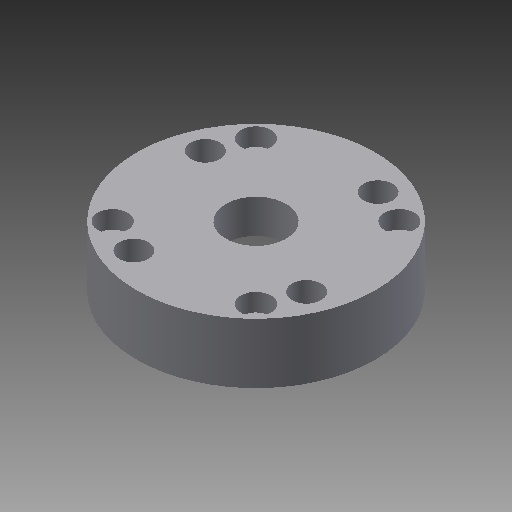
# Autodesk Inventor part: 09-1NT-0.125-FO1_BM_heads-bif
Saved by Autodesk Inventor 2019.4 (Build 234330000, 330)
## iProperties
Category: PARTsolutions
Company: BIMBA
Created: 2020-02-04
Part Number: 09-1NT-0.125-FO1_BM_heads-bif
Material: Generic
Catalog Web Link: www.cadenas.de
Description: FO1 Basic Model Heads-Bimba FLAT-1
Vendor: BIMBA
Document SubType Name: Modeling
Designer: psadmin
Manufacturer: BIMBA
Mass: 18.4876 g
Surface Area: 81.253 cm^2
Volume: 18.4876 cm^3
Density: 1 g/cm^3
Appearance: PSOLRGB-211-211-211
PSOL_IDENT_0: {$CADENAS_DATA\23d-libs\bimba\bimba_brand\bimba_imperial\bimba_full_line\flat_cylinders\fo1\fo1_basi
PSOL_IDENT_1: c_model_heads_right.prj},268 {VTYP=3D},{NB=09-1NT-0.125-FO1_BM_heads-bif},{LINA=09-1NT-0.125-FO1_BM_
PSOL_IDENT_2: heads-bif},{NN=FO1 Basic Model Heads},{DATE=22.01.2020 09:06:03},{GEOMDATE=10.10.2019 07:16:13},{VER
PSOL_IDENT_3: SION=},{LINEID=30},{WBVAR=MNT,LRR,ER,RTX,HD,STPT1,STPT2,STPT3,STPT4,PP,MRS,RL1},{WBNUMERIC=RL1}  {NB=
PSOL_IDENT_4: 09-1NT-0.125-FO1_BM_heads-bif},{LINA=09-1NT-0.125-FO1_BM_heads-bif},{KT=DUMMY},{PN=09-1NT-0.125-FO1_
PSOL_IDENT_5: BM_heads},{BORE=1.06250000},{BOREPN=09},{MNT=},{MNTALG='','Standard Counterbored Mounting Holes','1'
PSOL_IDENT_6: ,'Pivot Mount','1N','Pivot Mount 90 Deg. from Standard','2','[2] Trunnion Mount','3R','Threaded Moun
PSOL_IDENT_7: ting Holes, Rear','4R','Screw Clearance Holes, Rear','5','Front Nose Mount [5]','6','F Series Interc
PSOL_IDENT_8: hange, Counterbored, Rear [6]' ,'7R','F Series Interchange, Threaded, Rear [7R]'},{LRR=1},{ER=},{RTX=
PSOL_IDENT_9: NT},{RTXALG='', 'Standard', 'CFT', 'Coarse Female Thread', 'CMT'  , 'Male Rod Thread (Coarse)','MT',
PSOL_IDENT_10: 'Male Rod End (Fine)', 'NT'  , 'Non-Threaded Rod'},{HD=},{STPT1=},{STPT2=},{STPT3=},{STPT4=},{PP=},
PSOL_IDENT_11: {MRS=},{PPALG='','Standard','P2','Port Position #2','P3','Port Position #3','P4','Port Position #4'}
PSOL_IDENT_12: ,{A=1.98800000},{C=1.68800000},{AR=1.69000000},{DD=4.00000000},{D=0.13800000},{CPIL=0.15600000},{DC=
PSOL_IDENT_13: 0.25000000},{DCP=0.14800000},{DCD=1.68700000},{ES=0.31250000},{EC=0.31250000},{ED=0.70000000},{F=0.5
PSOL_IDENT_14: 0000000},{H=0.44000000},{J=0.5},{J1=0.50000000},{K=0.28},{K1=0.28000000},{K2=0.44000000},{L=0.405000
PSOL_IDENT_15: 00},{LDP=0.35500000},{LP=0.12500000},{LPDP=0.51000000},{TD=1.12200000},{TDDP=0.21800},{LSF=0.0000000
PSOL_IDENT_16: 0},{LSFDP=0.00000000},{AA=0.13000000},{AB=1.50000000},{AC=0.75000000},{AD=1.00000000},{AD1=UNS},{AE=
PSOL_IDENT_17: 0.99750000},{AF=0.55000000},{M=0.50000000},{N=0.25000000},{P=0.25000000},{Q=0.19000000},{QQ=0.252},{
PSOL_IDENT_18: R=0.13800000},{S=0.37500000},{T=0.25000000},{U=0.25000000},{W=0.81200000},{X=0.25000000},{Y=0.750000
PSOL_IDENT_19: 00},{Z=0.19000000},{A13=0.13800000},{A14=0.25000000},{ANGLE=45.00000000},{JY=0.5},{JH=0.5},{PANGLE=0
PSOL_IDENT_20: },{ANGLE1=67.5},{ANGLE11=67.50000000},{D11=0.156},{CONX=0.25000000},{CONY=0.20000000},{G=0.07000000}
PSOL_IDENT_21: ,{HH=0.55000000},{RD=0.27200000},{HDADD1=0.19000000},{HDADD=0},{GW=0.1095},{GD=0.8905},{GR=0.0460},{
PSOL_IDENT_22: PW=0.1300},{PD=0.9975},{PR=0.0150},{RL1=0.12500},{CS=1.55600},{DS=0.15400},{DCS=0.24200},{DCSP=0.180
PSOL_IDENT_23: 00},{C4=1.68800},{CD=1.68800},{C6=1.68800},{D6=0.20400},{DC6=0.37500},{DC6P=0.20000},{C7=1.68800},{R
PSOL_IDENT_24: 7=0.19000},{RC=1.55600},{RT=0.138},{RCB=0.15000},{RCD=0.10000},{PB1=0.000},{PB2=0.0000},{JB=0.302},{
PSOL_IDENT_25: AP=1.9900},{PCB=0.2500},{PCD=0.1560},{PCBD=0.145},{ALPH=65},{BDIA=0.900},{BD=0.058},{MNTRG=},{L5=1.2
PSOL_IDENT_26: 50},{NDM5=1.000},{A5=0.13000},{NANG=22.5},{UNANG=7.500}
NN: FO1 Basic Model Heads
NT: Bimba FLAT-1
NB: 09-1NT-0.125-FO1_BM_heads-bif
NBSYN: $PN.-bif
LINA: 09-1NT-0.125-FO1_BM_heads-bif
PN: 09-1NT-0.125-FO1_BM_heads
BORE: 0
BOREPN: 09
MNT: Standard Counterbored Mounting Holes
LRR: 1
ER: Single Rod
RTX: Non-Threaded Rod
HD: Standard Rear Head
STPT1: Without T1
STPT2: Without T2
STPT3: Without T3
STPT4: Without T4
PP: Standard
MRS: Without -Z
A: 1.988
C: 1.688
AR: 1.69
DD: 4
D: 0.138
CPIL: 0.156
DC: 0.25
DCP: 0.148
DCD: 1.687
ES: 0.3125
EC: 0.3125
ED: 0.7
F: 0.5
H: 0.44
J1: 0.5
K1: 0.28
K2: 0.44
L: 0.405
LDP: 0.355
LP: 0.125
LPDP: 0.51
TD: 1.122
TDDP: 0.218
LSF: 0
LSFDP: 0
AA: 0.13
AB: 1.5
AC: 0.75
AD: 1
AD1: UNS
AE: 0.9975
AF: 0.55
M: 0.5
N: 0.25
P: 0.25
Q: 0.19
QQ: 0.252
R: 0.138
S: 0.375
T: 0.25
U: 0.25
W: 0.812
X: 0.25
Y: 0.75
Z: 0.19
A13: 0.138
A14: 0.25
ANGLE: 45
ANGLE11: 67.5
CONX: 0.25
CONY: 0.2
G: 0.07
HH: 0.55
RD: 0.272
HDADD1: 0.19
GW: 0.1095
GD: 0.8905
GR: 0.046
PW: 0.13
PD: 0.9975
PR: 0.015
RL1: 0.125
CS: 1.556
DS: 0.154
DCS: 0.242
DCSP: 0.18
C4: 1.688
C6: 1.688
D6: 0.204
DC6: 0.375
DC6P: 0.2
C7: 1.688
R7: 0.19
RC: 1.556
RT: 0.138
RCB: 0.15
RCD: 0.1
PB1: 0
PB2: 0
AP: 1.99
PCB: 0.25
PCD: 0.156
PCBD: 0.145
BDIA: 0.9
BD: 0.058
L5: 1.25
NDM5: 1
A5: 0.13
NANG: 22.5
UNANG: 7.5
SUPPLIER: BIMBA
ARTICLENO: 09-1NT-0.125-FO1_BM_heads-bif
BOMINFO: 09-1NT-0.125-FO1_BM_heads-bif
CREATOR: CADENAS GmbH
Title: 09-1NT-0.125-FO1_BM_heads-bif
Author: Cadenas PARTsolutions
Comments: Bimba FLAT-1
Autodesk Inventor part; units mm, degrees
sketch "Sketch_1" plane through (0, 0, 0) normal (0, 0, 1) x (1, 0, 0)
  line L0 (0, 0) -> (0, 12.7)
  line L1 (0, 12.7) -> (25.2476, 12.7)
  line L2 (25.2476, 12.7) -> (25.2476, 0)
  line L3 (25.2476, 0) -> (0, 0)
  line L4 (0, 0) -> (0, 12.7)
  constraints: 10 end point
revolve "Revolution1" add sketch "Sketch_1" angle 360 about axis through (0, 0, 0) along (0, -1, 0)
sketch "Sketch_84" plane through (0, 0, 0) normal (0, 0, 1) x (1, 0, 0)
  line L0 (-16.2306, 5.588) -> (-25.2476, 5.588)
  line L1 (-25.2476, 5.588) -> (-25.2476, 11.0427)
  line L2 (-25.2476, 11.0427) -> (-24.6126, 10.4077)
  line L3 (-24.6126, 10.4077) -> (-16.2306, 10.146)
  line L4 (-16.2306, 10.146) -> (-16.2306, 5.588)
  line L5 (-16.2306, 5.588) -> (-25.2476, 5.588)
  constraints: 12 end point
revolve "Revolution2" cut sketch "Sketch_84" angle 360 about axis through (-16.2306, 5.588, 0) along (1, 0, 0)
thread "Thread1" size "1/8" designation "1/8 - 27 NPT" standard "NPT" full length
sketch "Sketch_85" plane through (0, 0, 0) normal (0, 0, 1) x (1, 0, 0)
  line L0 (-12.2936, 7.6708) -> (-25.2476, 7.6708)
  line L1 (-25.2476, 7.6708) -> (-25.2476, 9.2583)
  line L2 (-25.2476, 9.2583) -> (-13.2101, 9.2583)
  line L3 (-13.2101, 9.2583) -> (-12.2936, 7.6708)
  line L4 (-12.2936, 7.6708) -> (-25.2476, 7.6708)
  constraints: 10 end point
revolve "Revolution3" cut sketch "Sketch_85" angle 360 about axis through (-12.2936, 7.6708, 0) along (1, 0, 0)
sketch "Sketch4" plane through (0, 12.7, 0) normal (0, 1, 0) x (1, 0, 0)
  point P0 (-15.1587, 15.1587)
hole "Hole1" at (-15.1587, 12.7, -15.1587) direction (0, -1, 0) diameter 3.9624 depth 12.7 counterbore diameter 6.35 counterbore depth 3.7592
sketch "Sketch5" plane through (0, 12.7, 0) normal (0, 1, 0) x (1, 0, 0)
  point P0 (-15.1587, -15.1587)
hole "Hole2" at (-15.1587, 12.7, 15.1587) direction (0, -1, 0) diameter 3.9624 depth 12.7 counterbore diameter 6.35 counterbore depth 3.7592
sketch "Sketch6" plane through (0, 12.7, 0) normal (0, 1, 0) x (1, 0, 0)
  point P0 (15.1587, -15.1587)
hole "Hole3" at (15.1587, 12.7, 15.1587) direction (0, -1, 0) diameter 3.9624 depth 12.7 counterbore diameter 6.35 counterbore depth 3.7592
sketch "Sketch7" plane through (0, 12.7, 0) normal (0, 1, 0) x (1, 0, 0)
  point P0 (15.1587, 15.1587)
hole "Hole4" at (15.1587, 12.7, -15.1587) direction (0, -1, 0) diameter 3.9624 depth 12.7 counterbore diameter 6.35 counterbore depth 3.7592
sketch "Sketch8" plane through (0, 0, 0) normal (0, -1, 0) x (1, 0, 0)
  point P0 (0, 0)
hole "Hole5" at (0, 0, 0) direction (0, 1, 0) diameter 12.7508 depth 12.7
sketch "Sketch_9" plane through (0, 0, 0) normal (0, 0, 1) x (1, 0, 0)
  line L0 (0, 0) -> (0, 5.5372)
  line L1 (0, 5.5372) -> (14.2494, 5.5372)
  line L2 (14.2494, 5.5372) -> (14.2494, 0)
  line L3 (14.2494, 0) -> (0, 0)
  line L4 (0, 0) -> (0, 5.5372)
  constraints: 10 end point
revolve "Revolution4" cut sketch "Sketch_9" angle 360 about axis through (0, 0, 0) along (0, -1, 0)
sketch "Sketch10" plane through (0, 12.7, 0) normal (0, 1, 0) x (1, 0, 0)
  point P0 (-18.257, 7.5623)
hole "Hole6" at (-18.257, 12.7, -7.5623) direction (0, -1, 0) diameter 3.9116 depth 12.7 counterbore diameter 6.1468 counterbore depth 4.572
pattern_linear "Rectangular Pattern1" count 2 spacing 27.9466 along (0.9239, 0, -0.3827) count 2 spacing 27.9466 along (0.3827, 0, 0.9239) of "Hole6"
ref_plane "a1_XY" through (0, 12.7, -25.2476) normal (0, 1, 0) x (1, 0, 0)
ref_plane "a1_YZ" through (0, 12.7, -25.2476) normal (1, 0, 0) x (0, 0, -1)
ref_plane "a1_ZX" through (0, 12.7, -25.2476) normal (0, 0, -1) x (0, 1, 0)
ref_plane "a2_XY" through (0, 12.7, 25.2476) normal (0, 1, 0) x (1, 0, 0)
ref_plane "a2_YZ" through (0, 12.7, 25.2476) normal (1, 0, 0) x (0, 0, -1)
ref_plane "a2_ZX" through (0, 12.7, 25.2476) normal (0, 0, -1) x (0, 1, 0)
ref_plane "ab_tr1_XY" through (-12.9439, 0, -1.7041) normal (0, 1, 0) x (1, 0, 0)
ref_plane "ab_tr1_YZ" through (-12.9439, 0, -1.7041) normal (1, 0, 0) x (0, 0, -1)
ref_plane "ab_tr1_ZX" through (-12.9439, 0, -1.7041) normal (0, 0, -1) x (0, 1, 0)
ref_plane "ab_tr2_XY" through (12.9439, 0, 1.7041) normal (0, 1, 0) x (1, 0, 0)
ref_plane "ab_tr2_YZ" through (12.9439, 0, 1.7041) normal (1, 0, 0) x (0, 0, -1)
ref_plane "ab_tr2_ZX" through (12.9439, 0, 1.7041) normal (0, 0, -1) x (0, 1, 0)
ref_plane "ab_tr3_XY" through (-1.7041, 0, 12.9439) normal (0, 1, 0) x (1, 0, 0)
ref_plane "ab_tr3_YZ" through (-1.7041, 0, 12.9439) normal (1, 0, 0) x (0, 0, -1)
ref_plane "ab_tr3_ZX" through (-1.7041, 0, 12.9439) normal (0, 0, -1) x (0, 1, 0)
ref_plane "ab_tr4_XY" through (1.7041, 0, -12.9439) normal (0, 1, 0) x (1, 0, 0)
ref_plane "ab_tr4_YZ" through (1.7041, 0, -12.9439) normal (1, 0, 0) x (0, 0, -1)
ref_plane "ab_tr4_ZX" through (1.7041, 0, -12.9439) normal (0, 0, -1) x (0, 1, 0)
ref_plane "ar3_XY" through (-8.2135, 5.5372, 19.8292) normal (0, 1, 0) x (1, 0, 0)
ref_plane "ar3_YZ" through (-8.2135, 5.5372, 19.8292) normal (1, 0, 0) x (0, 0, -1)
ref_plane "ar3_ZX" through (-8.2135, 5.5372, 19.8292) normal (0, 0, -1) x (0, 1, 0)
ref_plane "ar4_XY" through (19.8292, 5.5372, 8.2135) normal (0, 1, 0) x (1, 0, 0)
ref_plane "ar4_YZ" through (19.8292, 5.5372, 8.2135) normal (1, 0, 0) x (0, 0, -1)
ref_plane "ar4_ZX" through (19.8292, 5.5372, 8.2135) normal (0, 0, -1) x (0, 1, 0)
ref_plane "ar5_XY" through (8.2135, 5.5372, -19.8292) normal (0, 1, 0) x (1, 0, 0)
ref_plane "ar5_YZ" through (8.2135, 5.5372, -19.8292) normal (1, 0, 0) x (0, 0, -1)
ref_plane "ar5_ZX" through (8.2135, 5.5372, -19.8292) normal (0, 0, -1) x (0, 1, 0)
ref_plane "ar6_XY" through (-19.8292, 5.5372, -8.2135) normal (0, 1, 0) x (1, 0, 0)
ref_plane "ar6_YZ" through (-19.8292, 5.5372, -8.2135) normal (1, 0, 0) x (0, 0, -1)
ref_plane "ar6_ZX" through (-19.8292, 5.5372, -8.2135) normal (0, 0, -1) x (0, 1, 0)
ref_plane "b1_XY" through (0, 12.7, 0) normal (0, 1, 0) x (1, 0, 0)
ref_plane "b1_YZ" through (0, 12.7, 0) normal (1, 0, 0) x (0, 0, -1)
ref_plane "b1_ZX" through (0, 12.7, 0) normal (0, 0, -1) x (0, 1, 0)
ref_plane "c11_XY" through (-15.1587, 12.7, -15.1587) normal (0, 1, 0) x (1, 0, 0)
ref_plane "c11_YZ" through (-15.1587, 12.7, -15.1587) normal (1, 0, 0) x (0, 0, -1)
ref_plane "c11_ZX" through (-15.1587, 12.7, -15.1587) normal (0, 0, -1) x (0, 1, 0)
ref_plane "c22_XY" through (15.1587, 12.7, 15.1587) normal (0, 1, 0) x (1, 0, 0)
ref_plane "c22_YZ" through (15.1587, 12.7, 15.1587) normal (1, 0, 0) x (0, 0, -1)
ref_plane "c22_ZX" through (15.1587, 12.7, 15.1587) normal (0, 0, -1) x (0, 1, 0)
ref_plane "d11_XY" through (-16.5596, 12.7, -13.7578) normal (0, 1, 0) x (1, 0, 0)
ref_plane "d11_YZ" through (-16.5596, 12.7, -13.7578) normal (1, 0, 0) x (0, 0, -1)
ref_plane "d11_ZX" through (-16.5596, 12.7, -13.7578) normal (0, 0, -1) x (0, 1, 0)
ref_plane "d22_XY" through (-13.7578, 12.7, -16.5596) normal (0, 1, 0) x (1, 0, 0)
ref_plane "d22_YZ" through (-13.7578, 12.7, -16.5596) normal (1, 0, 0) x (0, 0, -1)
ref_plane "d22_ZX" through (-13.7578, 12.7, -16.5596) normal (0, 0, -1) x (0, 1, 0)
ref_plane "j_XY" through (0, 0, 0) normal (0, 1, 0) x (1, 0, 0)
ref_plane "j_YZ" through (0, 0, 0) normal (1, 0, 0) x (0, 0, -1)
ref_plane "j_ZX" through (0, 0, 0) normal (0, 0, -1) x (0, 1, 0)
ref_plane "k1_XY" through (-25.2476, 5.588, 0) normal (0, 0, 1) x (1, 0, 0)
ref_plane "k1_YZ" through (-25.2476, 5.588, 0) normal (1, 0, 0) x (0, 1, 0)
ref_plane "k1_ZX" through (-25.2476, 5.588, 0) normal (0, 1, 0) x (0, 0, 1)
ref_plane "k2_XY" through (-25.2476, 12.7, 0) normal (0, 0, 1) x (1, 0, 0)
ref_plane "k2_YZ" through (-25.2476, 12.7, 0) normal (1, 0, 0) x (0, 1, 0)
ref_plane "k2_ZX" through (-25.2476, 12.7, 0) normal (0, 1, 0) x (0, 0, 1)
ref_plane "nut_XY" through (0, 26.9875, 0) normal (0, 1, 0) x (1, 0, 0)
ref_plane "nut_YZ" through (0, 26.9875, 0) normal (1, 0, 0) x (0, 0, -1)
ref_plane "nut_ZX" through (0, 26.9875, 0) normal (0, 0, -1) x (0, 1, 0)
ref_plane "po1_XY" through (18.257, 0, 7.5623) normal (0, 1, 0) x (1, 0, 0)
ref_plane "po1_YZ" through (18.257, 0, 7.5623) normal (1, 0, 0) x (0, 0, -1)
ref_plane "po1_ZX" through (18.257, 0, 7.5623) normal (0, 0, -1) x (0, 1, 0)
ref_plane "po2_XY" through (7.5623, 0, -18.257) normal (0, 1, 0) x (1, 0, 0)
ref_plane "po2_YZ" through (7.5623, 0, -18.257) normal (1, 0, 0) x (0, 0, -1)
ref_plane "po2_ZX" through (7.5623, 0, -18.257) normal (0, 0, -1) x (0, 1, 0)
ref_plane "po3_XY" through (-18.257, 0, -7.5623) normal (0, 1, 0) x (1, 0, 0)
ref_plane "po3_YZ" through (-18.257, 0, -7.5623) normal (1, 0, 0) x (0, 0, -1)
ref_plane "po3_ZX" through (-18.257, 0, -7.5623) normal (0, 0, -1) x (0, 1, 0)
ref_plane "po4_XY" through (-7.5623, 0, 18.257) normal (0, 1, 0) x (1, 0, 0)
ref_plane "po4_YZ" through (-7.5623, 0, 18.257) normal (1, 0, 0) x (0, 0, -1)
ref_plane "po4_ZX" through (-7.5623, 0, 18.257) normal (0, 0, -1) x (0, 1, 0)
ref_plane "r7_XY" through (2.413, 12.7, 21.4376) normal (0, 1, 0) x (1, 0, 0)
ref_plane "r7_YZ" through (2.413, 12.7, 21.4376) normal (1, 0, 0) x (0, 0, -1)
ref_plane "r7_ZX" through (2.413, 12.7, 21.4376) normal (0, 0, -1) x (0, 1, 0)
ref_plane "r71_XY" through (0, 12.7, 21.4376) normal (0, 1, 0) x (1, 0, 0)
ref_plane "r71_YZ" through (0, 12.7, 21.4376) normal (1, 0, 0) x (0, 0, -1)
ref_plane "r71_ZX" through (0, 12.7, 21.4376) normal (0, 0, -1) x (0, 1, 0)
ref_plane "r72_XY" through (-2.413, 12.7, 21.4376) normal (0, 1, 0) x (1, 0, 0)
ref_plane "r72_YZ" through (-2.413, 12.7, 21.4376) normal (1, 0, 0) x (0, 0, -1)
ref_plane "r72_ZX" through (-2.413, 12.7, 21.4376) normal (0, 0, -1) x (0, 1, 0)
ref_plane "r73_XY" through (0, 12.7, -21.4376) normal (0, 1, 0) x (1, 0, 0)
ref_plane "r73_YZ" through (0, 12.7, -21.4376) normal (1, 0, 0) x (0, 0, -1)
ref_plane "r73_ZX" through (0, 12.7, -21.4376) normal (0, 0, -1) x (0, 1, 0)
ref_plane "rg_XY" through (0, 12.7, 0) normal (0, 1, 0) x (1, 0, 0)
ref_plane "rg_YZ" through (0, 12.7, 0) normal (1, 0, 0) x (0, 0, -1)
ref_plane "rg_ZX" through (0, 12.7, 0) normal (0, 0, -1) x (0, 1, 0)
ref_plane "rh_XY" through (0, 12.7, 0) normal (0, 1, 0) x (1, 0, 0)
ref_plane "rh_YZ" through (0, 12.7, 0) normal (1, 0, 0) x (0, 0, -1)
ref_plane "rh_ZX" through (0, 12.7, 0) normal (0, 0, -1) x (0, 1, 0)
ref_plane "rs_1_XY" through (-15.1587, 15.2908, -15.1587) normal (0, 1, 0) x (1, 0, 0)
ref_plane "rs_1_YZ" through (-15.1587, 15.2908, -15.1587) normal (1, 0, 0) x (0, 0, -1)
ref_plane "rs_1_ZX" through (-15.1587, 15.2908, -15.1587) normal (0, 0, -1) x (0, 1, 0)
ref_plane "rs_2_XY" through (-15.1587, 15.2908, 15.1587) normal (0, 1, 0) x (1, 0, 0)
ref_plane "rs_2_YZ" through (-15.1587, 15.2908, 15.1587) normal (1, 0, 0) x (0, 0, -1)
ref_plane "rs_2_ZX" through (-15.1587, 15.2908, 15.1587) normal (0, 0, -1) x (0, 1, 0)
ref_plane "rs_3_XY" through (15.1587, 15.2908, 15.1587) normal (0, 1, 0) x (1, 0, 0)
ref_plane "rs_3_YZ" through (15.1587, 15.2908, 15.1587) normal (1, 0, 0) x (0, 0, -1)
ref_plane "rs_3_ZX" through (15.1587, 15.2908, 15.1587) normal (0, 0, -1) x (0, 1, 0)
ref_plane "rs_4_XY" through (15.1587, 15.2908, -15.1587) normal (0, 1, 0) x (1, 0, 0)
ref_plane "rs_4_YZ" through (15.1587, 15.2908, -15.1587) normal (1, 0, 0) x (0, 0, -1)
ref_plane "rs_4_ZX" through (15.1587, 15.2908, -15.1587) normal (0, 0, -1) x (0, 1, 0)
ref_plane "sc1_XY" through (7.5623, 8.128, -18.257) normal (0, 1, 0) x (1, 0, 0)
ref_plane "sc1_YZ" through (7.5623, 8.128, -18.257) normal (1, 0, 0) x (0, 0, -1)
ref_plane "sc1_ZX" through (7.5623, 8.128, -18.257) normal (0, 0, -1) x (0, 1, 0)
ref_plane "sc2_XY" through (-18.257, 8.128, -7.5623) normal (0, 1, 0) x (1, 0, 0)
ref_plane "sc2_YZ" through (-18.257, 8.128, -7.5623) normal (1, 0, 0) x (0, 0, -1)
ref_plane "sc2_ZX" through (-18.257, 8.128, -7.5623) normal (0, 0, -1) x (0, 1, 0)
ref_plane "sc3_XY" through (-7.5623, 8.128, 18.257) normal (0, 1, 0) x (1, 0, 0)
ref_plane "sc3_YZ" through (-7.5623, 8.128, 18.257) normal (1, 0, 0) x (0, 0, -1)
ref_plane "sc3_ZX" through (-7.5623, 8.128, 18.257) normal (0, 0, -1) x (0, 1, 0)
ref_plane "sc4_XY" through (18.257, 8.128, 7.5623) normal (0, 1, 0) x (1, 0, 0)
ref_plane "sc4_YZ" through (18.257, 8.128, 7.5623) normal (1, 0, 0) x (0, 0, -1)
ref_plane "sc4_ZX" through (18.257, 8.128, 7.5623) normal (0, 0, -1) x (0, 1, 0)
ref_plane "to_dummy_XY" through (0, 12.7, 0) normal (0, 1, 0) x (1, 0, 0)
ref_plane "to_dummy_YZ" through (0, 12.7, 0) normal (1, 0, 0) x (0, 0, -1)
ref_plane "to_dummy_ZX" through (0, 12.7, 0) normal (0, 0, -1) x (0, 1, 0)
ref_plane "to_nut_XY" through (0, 16.002, 0) normal (0, 1, 0) x (1, 0, 0)
ref_plane "to_nut_YZ" through (0, 16.002, 0) normal (1, 0, 0) x (0, 0, -1)
ref_plane "to_nut_ZX" through (0, 16.002, 0) normal (0, 0, -1) x (0, 1, 0)
ref_plane "to_rod_XY" through (0, 0, 0) normal (0, 1, 0) x (1, 0, 0)
ref_plane "to_rod_YZ" through (0, 0, 0) normal (1, 0, 0) x (0, 0, -1)
ref_plane "to_rod_ZX" through (0, 0, 0) normal (0, 0, -1) x (0, 1, 0)
ref_plane "to_tube_XY" through (0, 5.5372, 0) normal (0, 1, 0) x (1, 0, 0)
ref_plane "to_tube_YZ" through (0, 5.5372, 0) normal (1, 0, 0) x (0, 0, -1)
ref_plane "to_tube_ZX" through (0, 5.5372, 0) normal (0, 0, -1) x (0, 1, 0)
ref_plane "to_wiper_XY" through (0, 12.7, 0) normal (0, 1, 0) x (1, 0, 0)
ref_plane "to_wiper_YZ" through (0, 12.7, 0) normal (1, 0, 0) x (0, 0, -1)
ref_plane "to_wiper_ZX" through (0, 12.7, 0) normal (0, 0, -1) x (0, 1, 0)
ref_plane "track1_XY" through (-13.0556, 0, 0) normal (0, 1, 0) x (1, 0, 0)
ref_plane "track1_YZ" through (-13.0556, 0, 0) normal (1, 0, 0) x (0, 0, -1)
ref_plane "track1_ZX" through (-13.0556, 0, 0) normal (0, 0, -1) x (0, 1, 0)
ref_plane "track2_XY" through (0, 0, -13.0556) normal (0, 1, 0) x (1, 0, 0)
ref_plane "track2_YZ" through (0, 0, -13.0556) normal (1, 0, 0) x (0, 0, -1)
ref_plane "track2_ZX" through (0, 0, -13.0556) normal (0, 0, -1) x (0, 1, 0)
ref_plane "track3_XY" through (13.0556, 0, 0) normal (0, 1, 0) x (1, 0, 0)
ref_plane "track3_YZ" through (13.0556, 0, 0) normal (1, 0, 0) x (0, 0, -1)
ref_plane "track3_ZX" through (13.0556, 0, 0) normal (0, 0, -1) x (0, 1, 0)
ref_plane "track4_XY" through (0, 0, 13.0556) normal (0, 1, 0) x (1, 0, 0)
ref_plane "track4_YZ" through (0, 0, 13.0556) normal (1, 0, 0) x (0, 0, -1)
ref_plane "track4_ZX" through (0, 0, 13.0556) normal (0, 0, -1) x (0, 1, 0)
body "Solid1"
